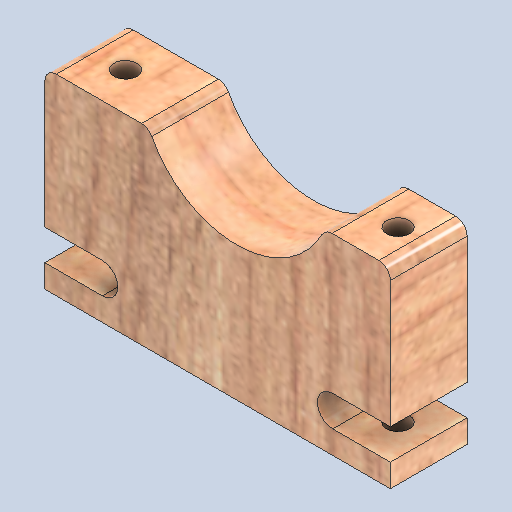
# Autodesk Inventor part: telo
Saved by Autodesk Inventor 2025.2 (Build 292293000, 293)
## iProperties
Created: 2025-04-28
Part Number: telo
Material: Wood (Birch)
Document SubType Name: Modeling
Designer: fanda
Density: 0.55 g/cm^3
Appearance: Birch - Natural Polished
Author: fanda
Autodesk Inventor part; units mm, degrees
ref_plane "YZ Plane" through (0, 0, 0) normal (1, 0, 0) x (0, 1, 0)
ref_plane "XZ Plane" through (0, 0, 0) normal (0, 1, 0) x (-1, 0, 0)
ref_plane "XY Plane" through (0, 0, 0) normal (0, 0, 1) x (1, 0, 0)
sketch "Sketch1" plane through (0, 0, 0) normal (0, 0, 1) x (1, 0, 0)
  line L0 (-9.5227, 1.8075) -> (80.4773, 1.8075)
  line L1 (80.4773, 1.8075) -> (80.4773, 7.8075)
  line L2 (80.4773, 7.8075) -> (65.4773, 7.8075)
  line L3 (65.4773, 15.8075) -> (80.4773, 15.8075)
  line L4 (80.4773, 15.8075) -> (80.4773, 48.8075)
  arc A0 (65.4773, 15.8075) -> (65.4773, 7.8075) centre (65.4773, 11.8075) ccw
  line L5 (77.4773, 51.8075) -> (65.2765, 51.8075)
  arc A1 (80.4773, 48.8075) -> (77.4773, 51.8075) centre (77.4773, 48.8075) ccw
  line L6 (-9.5227, 1.8075) -> (-9.5227, 7.8075)
  line L7 (-9.5227, 15.8075) -> (-9.5227, 48.8075)
  line L8 (-9.5227, 7.8075) -> (5.4773, 7.8075)
  line L9 (5.4773, 15.8075) -> (-9.5227, 15.8075)
  arc A2 (5.4773, 7.8075) -> (5.4773, 15.8075) centre (5.4773, 11.8075) ccw
  line L10 (-6.5227, 51.8075) -> (15.6781, 51.8075)
  arc A3 (-6.5227, 51.8075) -> (-9.5227, 48.8075) centre (-6.5227, 48.8075) ccw
  arc A4 (18.3351, 50.2003) -> (62.6194, 50.2003) centre (40.4773, 61.8075) ccw
  arc A5 (18.3351, 50.2003) -> (15.6781, 51.8075) centre (15.6781, 48.8075) ccw
  arc A6 (65.2765, 51.8075) -> (62.6194, 50.2003) centre (65.2765, 48.8075) ccw
  point P0 (0, 0)
  point P1 (80.4773, 51.8075)
  point P2 (63.3902, 51.8075)
  point P3 (17.5644, 51.8075)
  dimension "d0" = 90
  dimension "d1" = 6
  dimension "d2" = 15
  dimension "d3" = 8
  dimension "d4" = 36
  dimension "d7" = 3
  dimension "d8" = 6
  dimension "d16" = 50
  dimension "d17" = 3
  constraints: 22 end point, 16 point on circle, 7 centre point, 6 point on line, 6 tangent, 4 perpendicular, 2 horizontal, 1 equal radius
  measures "d0" distance of L0.start L0.end
  measures "d1" distance of L0.end L1.end
  measures "d2" distance of L1.end L2.end
  measures "d3" distance of L2.end L3.start
  measures "d4" distance of L3.end point (80.477, 51.807)
  measures "d7" radius of A1
  measures "d8" distance of L6.start L6.end
  measures "d16" diameter of A4
  measures "d17" radius of A5
extrude "Extrusion1" add sketch "Sketch1" along normal blind 20
sketch "Sketch2" plane through (-9.5227, 1.8075, 0) normal (0, -1, 0) x (1, 0, 0)
  line L0 (90, 0) -> (90, 20) projected
  circle A0 centre (82, 10) radius 3
  line L1 (3, 0) -> (3, 20) projected
  circle A1 centre (11, 10) radius 3
  point P0 (9.5227, 0)
  dimension "d21" = 6
  dimension "d23" = 6
  constraints: 2 centre point
  measures "d21" diameter of A0
  measures "d23" diameter of A1
extrude "Extrusion2" cut sketch "Sketch2" against normal blind 50
